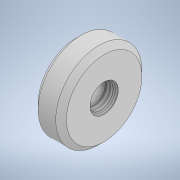
# Autodesk Inventor part: 711131
Saved by Autodesk Inventor 2022 (Build 260153000, 153)
## iProperties
Created: 2021-10-22
Part Number: 711131
Material: Типовые
Document SubType Name: Modeling
Designer: RaNSiD
Density: 1 g/cm^3
Appearance: По умолчанию
Mass: 22.5337 g
Surface Area: 51.5454 cm^2
Volume: 22.5337 cm^3
Author: RaNSiD
Autodesk Inventor part; units mm, degrees
ref_plane "YZ Plane" through (0, 0, 0) normal (1, 0, 0) x (0, 1, 0)
ref_plane "XZ Plane" through (0, 0, 0) normal (0, 1, 0) x (-1, 0, 0)
ref_plane "XY Plane" through (0, 0, 0) normal (0, 0, 1) x (1, 0, 0)
sketch "Эскиз1" plane through (-7.5, -11.4142, 0) normal (0, 0, 1) x (1, 0, 0)
  line L0 (0, 0) -> (0, 20)
  line L1 (0, 20) -> (2.8284, 22.8284)
  line L2 (0, 0) -> (15, 0)
  line L3 (15, 0) -> (15, 20)
  line L4 (15, 20) -> (12.1716, 22.8284)
  line L5 (12.1716, 22.8284) -> (2.8284, 22.8284)
  dimension "d5" = 20
  dimension "d4" = 4
  dimension "d3" = 135
  dimension "d2" = 15
  dimension "d1" = 4
  dimension "d0" = 135
  constraints: 12 end point, 1 horizontal, 1 parallel, 1 perpendicular, 1 vertical
  measures "d5" distance of L0.start L0.end
  measures "d4" distance of L0.end L1.end
  measures "d3" angle of L0 L1
  measures "d2" distance of L0.start L2.end
  measures "d1" distance of L3.end L4.end
  measures "d0" angle of L4 L3
revolve "Вращение1" add sketch "Эскиз1" angle 360 about axis through (-7.5, -11.4142, 0) along (1, 0, 0)
sketch "Эскиз2" plane through (7.5, -11.4142, 0) normal (1, 0, 0) x (0, 0, -1)
  circle A0 centre (0, 0) radius 20 construction
  point P0 (0, 11.4142)
  constraints: 1 coincident
hole "Отверстие1" at (7.5, -11.4142, 0) direction (-1, 0, 0) diameter 13 depth 6 tip angle 145 countersink diameter 15 countersink angle 60
thread "Резьба1" size "M14x2" class "6H" standard "ANSI Metric M Profile" full length
thread "Резьба2" size "Rc 1/16" standard "ISO Taper Internal" full length
